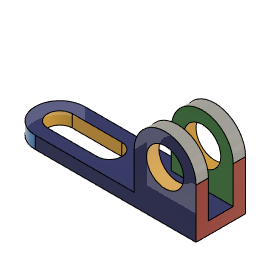
darshan_nair_exercise5 (Autodesk Fusion 360 design; units mm, degrees)
Autodesk Fusion 360 part; units mm, degrees
sketch "Sketch1" plane through (0, 0, 0) normal (0, 0, 1) x (1, 0, 0)
  line L0 (0, 0) -> (130, 0)
  line L1 (130, 0) -> (130, 40)
  line L2 (130, 40) -> (0, 40)
  line L3 (0, 40) -> (0, 0) construction
  arc A0 (0, 40) -> (0, 0) centre (0, 20) ccw
  arc A1 (0, 30) -> (0, 10) centre (0, 20) ccw
  line L4 (0, 30) -> (40, 30)
  line L5 (0, 10) -> (40, 10)
  arc A2 (40, 10) -> (39.9965, 30) centre (40, 20) ccw
  line L6 (-17.8729, 20) -> (60, 20) construction
  line L7 (40, 40) -> (40, 0) construction
  line L8 (130, 40) -> (80, 40)
  line L9 (80, 40) -> (80, 30)
  line L10 (80, 30) -> (130, 30)
  line L11 (130, 30) -> (130, 40)
  line L12 (130, 0) -> (80, 0)
  line L13 (80, 0) -> (80, 10)
  line L14 (80, 10) -> (130, 10)
  line L15 (130, 10) -> (130, 0)
  dimension "d1" = 130
  dimension "d2" = 40
  dimension "d3" = 20
  dimension "d4" = 40
  dimension "d5" = 40
  dimension "d6" = 50
  dimension "d7" = 10
  dimension "d8" = 50
  dimension "d9" = 10
  constraint horizontal L0
  constraint vertical L1
  constraint horizontal L2
  constraint vertical L3
  constraint coincident L0.start L3.end
  constraint midpoint L3 A0.centre
  constraint concentric A0 A1
  constraint coincident L3 A1.end
  constraint coincident L3 A1.start
  constraint perpendicular L3 L4
  constraint perpendicular L3 L5
  constraint coincident L4 A2.end
  constraint parallel L5 L6
  constraint coincident L2 L7.start
  constraint coincident L0 L7.end
  constraint perpendicular L0 L7
  constraint horizontal L8
  constraint vertical L9
  constraint horizontal L10
  constraint vertical L11
  constraint horizontal L12
  constraint vertical L13
  constraint horizontal L14
  constraint vertical L15
  measures "d1" distance of L0.start L0.end
  measures "d2" distance of L0.start L2.end
  measures "d3" diameter of A1
  measures "d4" distance of A1.start L4.end
  measures "d5" distance of A1.end L5.end
  measures "d6" distance of L1.end L8.end
  measures "d7" distance of L1.end L10.end
  measures "d8" distance of L0.end L12.end
  measures "d9" distance of L0.end L14.end
extrude "Extrude1" add sketch "Sketch1" along normal blind 10 contours L0 L1 L2 A0 L9 L10 L13 L14
sketch "Sketch2" plane through (0, 0, 0) normal (0, -1, 0) x (1, 0, 0)
  line L0 (0, 0) -> (80, 0)
  line L1 (80, 0) -> (80, 10)
  line L2 (80, 10) -> (0, 10)
  line L3 (0, 10) -> (0, 0)
  line L4 (80, 10) -> (80, 40)
  line L5 (80, 0) -> (130, 0)
  line L6 (130, 0) -> (130, 40)
  line L7 (80, 40) -> (130, 40) construction
  arc A0 (130, 40) -> (80, 40) centre (105, 40) ccw
  circle A1 centre (105, 40) radius 15
  dimension "d12" = 30
  dimension "d13" = 50
  dimension "d14" = 40
  dimension "d15" = 30
  constraint coincident L1.end L2.start
  constraint perpendicular L2 L4
  constraint coincident L0.end L1.start
  constraint perpendicular L1 L5
  constraint perpendicular L5 L6
  constraint tangent L6 A0
  constraint concentric A0 A1
  measures "d12" distance of L1.end L4.end
  measures "d13" distance of L0.end L5.end
  measures "d14" distance of L5.end L6.end
  measures "d15" diameter of A1
extrude "Extrude2" add sketch "Sketch2" against normal blind 10 contours L1 L4 L5 L6 A0
sketch "Sketch3" plane through (0, 30, 0) normal (0, 1, 0) x (-1, 0, 0)
  line L0 (-130, 0) -> (-80, 0)
  line L1 (-80, 0) -> (-80, 10)
  line L2 (-80, 10) -> (-130, 10)
  line L3 (-130, 10) -> (-130, 0)
  line L4 (-130, 10) -> (-130, 40)
  line L5 (-80, 10) -> (-80, 40)
  line L6 (-130, 40, -20) -> (-80, 40, -20)
  arc A0 (-80, 40) -> (-130, 40) centre (-105, 40) ccw
  circle A1 centre (-105, 40) radius 15
  point P0 (-130, 40)
  point P1 (-80, 40)
  dimension "d18" = 30
  dimension "d19" = 30
  dimension "d20" = 30
  constraint coincident L2.end L3.start
  constraint perpendicular L2 L4
  constraint coincident L1.end L2.start
  constraint perpendicular L2 L5
  constraint coincident P0 L4.end
  constraint coincident P1 L5.end
  constraint concentric A0 A1
  measures "d18" distance of L2.end P0
  measures "d19" distance of L1.end P1
  measures "d20" diameter of A1
extrude "Extrude3" add sketch "Sketch3" along normal blind 10 contours L0 L1 L2 L3
extrude "Extrude4" add sketch "Sketch3" along normal blind 10 contours L2 L4 L5 A0
sketch "Sketch4" plane through (0, 0, 0) normal (0, 0, 1) x (1, 0, 0)
  point P0 (130, 40)
  point P1 (0, 40)
  point P2 (130, 0)
  point P3 (80, 0)
  point P4 (130, 30)
  point P5 (130, 10)
  dimension "d25" = 130
  dimension "d26" = 50
  dimension "d27" = 20
  dimension "d28" = 10
  dimension "d29" = 10
  measures "d25" distance of P0 P1
  measures "d26" distance of P2 P3
  measures "d27" distance of P4 P5
  measures "d28" distance of P0 P4
  measures "d29" distance of P2 P5
sketch "Sketch5" plane through (0, 0, 0) normal (0, -1, 0) x (1, 0, 0)
  circle A0 centre (105, 40) radius 15
  line L0 (0, 0) -> (130, 0)
  line L1 (130, 0) -> (130, 40)
  arc A1 (130, 40) -> (80, 40) centre (105, 40) ccw
  line L2 (80, 40) -> (80, 10)
  line L3 (80, 10) -> (0, 10)
  line L4 (0, 10) -> (0, 0)
  point P0 (130, 0)
  dimension "d30" = 30
  dimension "d31" = 130
  measures "d30" distance of A1.end L2.end
  measures "d31" distance of P0 L0.start
sketch "Sketch6" plane through (130, 0, 0) normal (1, 0, 0) x (0, 1, 0)
  line L0 (0, 0) -> (40, 0)
  line L1 (40, 0) -> (40, 40)
  line L2 (40, 40) -> (30, 40)
  line L3 (30, 40) -> (30, 10)
  line L4 (30, 10) -> (10, 10)
  line L5 (10, 10) -> (10, 40)
  line L6 (10, 40) -> (0, 40)
  line L7 (0, 40) -> (0, 0)
  point P0 (10, 40)
  dimension "d32" = 10
  dimension "d33" = 10
  dimension "d34" = 40
  dimension "d35" = 40
  measures "d32" distance of L6.end P0
  measures "d33" distance of L1.end L2.end
  measures "d34" distance of L0.start L0.end
  measures "d35" distance of L0.end L1.end
